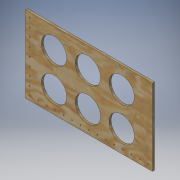
# Autodesk Inventor part: Bottom
Saved by Autodesk Inventor 2016 (Build 200138000, 138)
## iProperties
Created: 2016-01-30
Part Number: Bottom
Material: Generic
Document SubType Name: Modeling
Designer: ares-b02
Density: 1 g/cm^3
Appearance: Plywood - Weathered
Author: ares-b02
Autodesk Inventor part; units mm, degrees
ref_plane "YZ Plane" through (0, 0, 0) normal (1, 0, 0) x (0, 1, 0)
ref_plane "XZ Plane" through (0, 0, 0) normal (0, 1, 0) x (-1, 0, 0)
ref_plane "XY Plane" through (0, 0, 0) normal (0, 0, 1) x (1, 0, 0)
sketch "Sketch1" plane through (0, 0, 0) normal (0, 0, 1) x (1, 0, 0)
  line L0 (-206.3501, 165.9986) -> (174.6499, 165.9986)
  line L1 (174.6499, 165.9986) -> (174.6499, -63.9984)
  line L2 (174.6499, -63.9984) -> (-206.3501, -63.9984)
  line L3 (-206.3501, -63.9984) -> (-206.3501, 165.9986)
  point P0 (0, 0)
  dimension "d0" = 381
  dimension "d1" = 229.997
  constraints: 8 end point, 2 parallel, 1 horizontal, 1 perpendicular
  measures "d0" distance of L1.end L2.end
  measures "d1" distance of L0.end L1.end
extrude "Extrusion1" add sketch "Sketch1" along normal blind 6.35
hole "Hole1" at (-120.6251, 102.4986, 6.35) direction (0, 0, -1) diameter 76.2 end through all
pattern_linear "Rectangular Pattern1" count 3 spacing 101.6 along (1, 0, 0) count 2 spacing 101.6 along (0, -1, 0) of "Hole1"
hole "Hole2" at (-193.6501, -51.2984, 6.35) direction (0, 0, -1) diameter 3.175 end through all
pattern_linear "Rectangular Pattern2" count 14 spacing 25.4 along (1, 0, 0) of "Hole2"
hole "Hole3" at (161.9499, -51.2984, 6.35) direction (0, 0, -1) diameter 3.175 end through all
pattern_linear "Rectangular Pattern3" count 9 spacing 25.4 along (0, 1, 0) of "Hole2"
body "Solid1"
